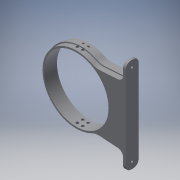
# Autodesk Inventor part: socketBracket
Saved by Autodesk Inventor 2016 (Build 200138000, 138)
## iProperties
Created: 2015-11-22
Part Number: socketBracket
Material: Generic
Document SubType Name: Modeling
Designer: Artur
Density: 1 g/cm^3
Appearance: Default
Author: Artur
Autodesk Inventor part; units mm, degrees
ref_plane "YZ Plane" through (0, 0, 0) normal (1, 0, 0) x (0, 1, 0)
sketch "Sketch1" plane through (0, 0, 0) normal (0, 1, 0) x (-1, 0, 0)
  circle A0 centre (0, 0) radius 60
  arc A1 (-28.3654, -56.2531) -> (-28.3654, 56.2531) centre (0, 0) ccw
  line L0 (-34.8246, 52.5) -> (0, 0) construction
  line L1 (0, 0) -> (-34.8246, -52.5) construction
  line L2 (0, 0) -> (-98.6538, 0) construction
  line L3 (-34.8246, 52.5) -> (-34.8246, -52.5) construction
  line L4 (-92, 88) -> (-92, -88)
  line L5 (-92, -88) -> (-87, -88)
  line L6 (-87, -88) -> (-87, -65.3517)
  line L7 (-92, 88) -> (-87, 88)
  line L8 (-87, 88) -> (-87, 65.3517)
  line L9 (-43.8806, 53.1075) -> (-77.6693, 55.3741)
  line L10 (-77.6693, -55.3741) -> (-43.8806, -53.1075)
  arc A2 (-87, 65.3517) -> (-77.6693, 55.3741) centre (-77, 65.3517) ccw
  arc A3 (-77.6693, -55.3741) -> (-87, -65.3517) centre (-77, -65.3517) ccw
  arc A4 (-43.8806, 53.1075) -> (-28.3654, 56.2531) centre (-41.8727, 83.0402) ccw
  arc A5 (-28.3654, -56.2531) -> (-43.8806, -53.1075) centre (-41.8727, -83.0402) ccw
  point P0 (-60, 0)
  point P1 (-92, 0)
  point P2 (-87, -56)
  point P3 (-87, 56)
  dimension "d0" = 120
  dimension "d1" = 63
  dimension "d2" = 105
  dimension "d3" = 32
  dimension "d4" = 176
  dimension "d5" = 5
  dimension "d6" = 5
  dimension "d7" = 32
  dimension "d8" = 32
  dimension "d9" = 10
  dimension "d10" = 10
  dimension "d11" = 30
  dimension "d12" = 30
  constraints: 22 end point, 13 point on circle, 8 point on line, 8 tangent, 5 centre point, 3 horizontal, 2 coincident, 2 perpendicular, 2 vertical, 1 horizontal alignment, 1 midpoint, 2 other
  measures "d1" radius of A1
  measures "d2" distance of L1.end L0.start
  measures "d3" distance from line of L4 point (-60, 0)
  measures "d4" distance of L4.start L4.end
  measures "d5" distance of L4.end L5.end
  measures "d6" distance of L4.start L7.end
  measures "d7" distance of L7.end point (-87, 56)
  measures "d8" distance of L5.end point (-87, -56)
  measures "d9" radius of A2
  measures "d10" radius of A3
  measures "d11" radius of A4
  measures "d12" radius of A5
extrude "Extrusion1" add sketch "Sketch1" along normal blind 24
sketch "Sketch2" plane through (92, 0, 88) normal (1, 0, 0) x (0, 0, -1)
  circle A0 centre (12, 12) radius 2
  line L0 (0, 0) -> (0, 24) construction
  line L1 (0, 12) -> (176, 12) construction
  line L2 (176, 0) -> (176, 24) construction
  line L3 (88, 12) -> (88, 46.8122) construction
  circle A1 centre (164, 12) radius 2
  point P0 (88, 0)
  dimension "d15" = 4
  dimension "d35" = 152
  constraints: 4 end point, 3 midpoint, 2 centre point, 1 point on line, 1 symmetric about line, 1 vertical, 1 other
  measures "d15" diameter of A0
  measures "d35" distance of A1.centre A0.centre
extrude "Extrusion2" cut sketch "Sketch2" against normal blind 24
fillet "Fillet1" radius 10 4 edges at (89.5, 24, 88) (89.5, 0, 88) (89.5, 24, -88) (89.5, 0, -88)
ref_plane "Work Plane1" through (0, 12, 0) normal (0, 1, 0) x (1, 0, 0)
sketch "Sketch3" plane through (0, 12, 0) normal (0, 1, 0) x (1, 0, 0)
  arc A0 (28.3654, 56.2531) -> (28.3654, -56.2531) centre (0, 0) ccw projected
  arc A1 (28.3654, 56.2531) -> (43.8806, 53.1075) centre (41.8727, 83.0402) ccw projected
  line L0 (77.6693, 55.3741) -> (43.8806, 53.1075) projected
  arc A2 (77.6693, 55.3741) -> (87, 65.3517) centre (77, 65.3517) ccw projected
  line L1 (87, 78) -> (87, 65.3517) projected
  arc A3 (43.8806, -53.1075) -> (28.3654, -56.2531) centre (41.8727, -83.0402) ccw projected
  line L2 (43.8806, -53.1075) -> (77.6693, -55.3741) projected
  arc A4 (87, -65.3517) -> (77.6693, -55.3741) centre (77, -65.3517) ccw projected
  line L3 (87, -65.3517) -> (87, -78) projected
  line L4 (87, -88) -> (87, -78) projected
  line L5 (87, 78) -> (87, 88) projected
  arc A5 (43.7468, -55.103) -> (29.2659, -58.0389) centre (41.8727, -83.0402) ccw
  arc A6 (29.2659, 58.0389) -> (29.2659, -58.0389) centre (0, 0) ccw
  arc A7 (29.2659, 58.0389) -> (43.8806, 55.1123) centre (41.8727, 83.0402) ccw
  line L6 (43.8806, 55.1123) -> (83.5224, 57.7715)
  line L7 (43.7468, -55.103) -> (83.522, -57.7712)
  arc A8 (87, -65.3517) -> (77.6693, -55.3741) centre (77, -65.3517) ccw projected
  line L8 (43.8806, -53.1075) -> (43.7468, -55.103) construction
  line L9 (43.8806, 55.1123) -> (43.8806, 53.1075) construction
  dimension "d21" = 2
  constraints: 9 point on circle, 8 end point, 3 centre point, 2 parallel, 1 perpendicular, 1 vertical, 2 other
  measures "d21" radial gap between concentric circles of A0 A6
extrude "Extrusion3" add sketch "Sketch3" along normal mid plane 6
ref_plane "Work Plane2" through (0, 12, 65) normal (0, 0, 1) x (1, 0, 0)
sketch "Sketch4" plane through (0, 12, 65) normal (0, 0, 1) x (1, 0, 0)
  line L0 (-60, 12) -> (60, 12) construction
  line L1 (60, -12) -> (-60, -12) construction
  line L2 (0, 12) -> (0, -12) construction
  line L3 (-43.2925, 0) -> (51.6055, 0) construction
  point P0 (0, 0)
  point P1 (5, 5)
  point P2 (-5, 5)
  point P3 (5, -5)
  point P4 (-5, -5)
  dimension "d24" = 10
  dimension "d25" = 10
  dimension "d26" = 10
  dimension "d27" = 10
  constraints: 4 end point, 2 midpoint, 2 symmetric about line, 1 horizontal, 1 perpendicular, 1 point on line
  measures "d24" diameter of point (-5, 5) L3
  measures "d25" diameter of point (5, 5) L3
  measures "d26" distance of point (-5, 5) point (5, 5)
  measures "d27" diameter of point (-5, 5) L2
hole "Hole1" at (5, 17, 65) at (-5, 17, 65) at (-5, 7, 65) at (5, 7, 65) direction (0, 0, -1) diameter 5 end through all
equation "\"d6\" = d5"
equation "\"d8\" = d7"
equation "\"d25\" = d24"
equation "\"d27\" = d26"
body "Solid1"
